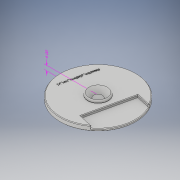
# Autodesk Inventor part: dissection_platform_v01
Saved by Autodesk Inventor 2019 (Build 230136000, 136)
## iProperties
Created: 2018-12-14
Part Number: dissection_platform_v01
Material: Generic
Document SubType Name: Modeling
Designer: Wilson Lab
Density: 1 g/cm^3
Appearance: Default
Author: Wilson Lab
Autodesk Inventor part; units mm, degrees
ref_plane "YZ Plane" through (0, 0, 0) normal (1, 0, 0) x (0, 1, 0)
ref_plane "XZ Plane" through (0, 0, 0) normal (0, 1, 0) x (-1, 0, 0)
ref_plane "XY Plane" through (0, 0, 0) normal (0, 0, 1) x (1, 0, 0)
sketch "Base Material Sketch" plane through (0, 0, 0) normal (0, 1, 0) x (-1, 0, 0)
  circle A0 centre (0, 0) radius 32.5
  dimension "d0" = 65
  constraints: 1 centre point, 1 coincident
  measures "d0" diameter of A0
extrude "Base Material Extrusion" add sketch "Base Material Sketch" along normal blind 4
sketch "Magnet Recess" plane through (0, 0, 0) normal (0, -1, 0) x (1, 0, 0)
  circle A0 centre (0, 0) radius 32.5 projected
  circle A1 centre (0, 27.5) radius 3.5
  line L0 (0, 0) -> (0, 32.5) construction
  circle A2 centre (0, 0) radius 32.5 construction
  circle A3 centre (-26.1541, 8.498) radius 3.5
  circle A4 centre (-16.1641, -22.248) radius 3.5
  circle A5 centre (16.1641, -22.248) radius 3.5
  circle A6 centre (26.1541, 8.498) radius 3.5
  dimension "d3" = 7
  dimension "d4" = 5
  dimension "d7" = 360
  constraints: 5 centre point, 2 end point, 1 point on line, 1 vertical, 1 vertical alignment, 12 other
  measures "d3" diameter of A1
  measures "d4" distance of A1.centre L0.end
extrude "Bottom Magnet Recess" cut sketch "Magnet Recess" against normal blind 1 contours A1 | A3 | A4 | A5 | A6
sketch "Central Well" plane through (0, 4, 0) normal (0, 1, 0) x (1, 0, 0)
  circle A0 centre (0, 0) radius 32.5 construction
  circle A1 centre (0, 0) radius 3.75
  dimension "d12" = 7.5
  constraints: 1 centre point, 1 coincident
  measures "d12" diameter of A1
extrude "Well Recess" cut sketch "Central Well" against normal blind 2
sketch "Sketch6" plane through (0, 4, 0) normal (0, 1, 0) x (1, 0, 0)
  circle A0 centre (0, 0) radius 7.75
  circle A1 centre (0, 0) radius 8.75
  dimension "d22" = 15.5
  dimension "d23" = 17.5
  constraints: 2 centre point, 2 coincident
  measures "d22" diameter of A0
  measures "d23" diameter of A1
extrude "Well Wall" add sketch "Sketch6" along normal blind 2
sketch "kimwipe recess sketch" plane through (0, 4, 0) normal (0, 1, 0) x (1, 0, 0)
  circle A0 centre (0, 0) radius 32.5 construction
  circle A1 centre (0, 0) radius 8.75 construction
  circle A2 centre (0, 0) radius 3.75 construction
  circle A3 centre (0, 0) radius 32.5 construction
  circle A4 centre (0, 0) radius 32.5 projected
  line L0 (16.9285, 17.1162) -> (55.4596, 8.4325)
  line L1 (55.4596, 8.4325) -> (46.4812, -31.4067)
  line L2 (46.4812, -31.4067) -> (7.95, -22.723)
  line L3 (7.95, -22.723) -> (16.9285, 17.1162)
  line L4 (16.9285, 17.1162) -> (46.4812, -31.4067) construction
  line L5 (55.4596, 8.4325) -> (7.95, -22.723) construction
  line L6 (0, 0) -> (12.4392, -2.8034) construction
  point P0 (31.7048, -7.1453)
  constraints: 14 end point, 3 midpoint, 2 parallel, 2 perpendicular, 1 coincident, 2 other
chamfer "Well Chamfer" distance 2 angle 45 2 edges at (-3.75, 4, 0) (-7.75, 4, 0)
fillet "Well Wall Fillet" radius 2 1 edges at (-8.75, 6, 0)
extrude "kimwipe recess" cut sketch "kimwipe recess sketch" against normal blind 2 contours A4 L2 L3 L0 | A4 L0 L1 L2 picked at (18.8525, -4.2886)
fillet "Aesthetic Filet" radius 0.5 14 edges at (12.6641, 0, -22.248) (-19.6641, 0, -22.248) (-29.6541, 0, 8.498) (-3.5, 0, 27.5) (22.6541, 0, 8.498) (32.5, 0, 0) (-7.3725, 4, -31.6527) (-14.1511, 4, 29.2574) (31.7048, 2, 7.1453) (12.4392, 4, 2.8034) (14.0633, 4, 24.1007) (20.1767, 3, 25.4785) (29.1551, 3, -14.3607) (23.0418, 4, -15.7384)
sketch "Sketch8" plane through (0, 4, 0) normal (0, 1, 0) x (-0.219854, 0, 0.9755328)
  line L0 (-23.8285, -62.331) -> (23.8285, -62.331) construction
  line L1 (23.8285, -62.331) -> (23.8285, 17.5) construction
  line L2 (23.8285, 17.5) -> (-23.8285, 17.5) construction
  line L3 (-23.8285, 17.5) -> (-23.8285, -62.331) construction
  circle A0 centre (0, 0) radius 17.5
  line L4 (-23.8285, 17.5) -> (23.8285, 17.5)
  line L5 (0, 0) -> (0, 17.5)
  line L6 (-14.128, -23.1128) -> (-14.3555, -23.1128)
  line L7 (-14.3555, -23.1128) -> (-14.3555, -22.9757)
  spline S0 degree 2 poles (-14.3555, -22.9757) (-14.408, -23.0194) (-14.4853, -23.0778) (-14.5378, -23.1026) knots 0 0 0 1 2 2 2
  spline S1 degree 2 poles (-14.5378, -23.1026) (-14.586, -23.1259) (-14.6895, -23.1507) (-14.7581, -23.1507) knots 0 0 0 1 2 2 2
  spline S2 degree 2 poles (-14.7581, -23.1507) (-14.869, -23.1507) (-15.0557, -23.0588) (-15.1213, -22.9698) knots 0 0 0 1 2 2 2
  spline S3 degree 2 poles (-15.1213, -22.9698) (-15.187, -22.8808) (-15.2599, -22.6183) (-15.2599, -22.4476) knots 0 0 0 1 2 2 2
  spline S4 degree 2 poles (-15.2599, -22.4476) (-15.2599, -22.2697) (-15.168, -22.01) (-15.0878, -21.9123) knots 0 0 0 1 2 2 2
  spline S5 degree 2 poles (-15.0878, -21.9123) (-15.0134, -21.8248) (-14.8048, -21.7241) (-14.6895, -21.7241) knots 0 0 0 1 2 2 2
  spline S6 degree 2 poles (-14.6895, -21.7241) (-14.5889, -21.7241) (-14.4387, -21.7693) (-14.3555, -21.816) knots 0 0 0 1 2 2 2
  line L8 (-14.3555, -21.816) -> (-14.3555, -21.2325)
  line L9 (-14.3555, -21.2325) -> (-14.128, -21.2325)
  line L10 (-14.128, -21.2325) -> (-14.128, -23.1128)
  line L11 (-14.3555, -22.7846) -> (-14.3555, -22.0042)
  spline S7 degree 2 poles (-14.3555, -22.0042) (-14.4401, -21.9633) (-14.5743, -21.9327) (-14.6516, -21.9327) knots 0 0 0 1 2 2 2
  spline S8 degree 2 poles (-14.6516, -21.9327) (-14.8267, -21.9327) (-15.025, -22.1953) (-15.025, -22.4432) knots 0 0 0 1 2 2 2
  spline S9 degree 2 poles (-15.025, -22.4432) (-15.025, -22.6825) (-14.8733, -22.9348) (-14.7056, -22.9348) knots 0 0 0 1 2 2 2
  spline S10 degree 2 poles (-14.7056, -22.9348) (-14.6166, -22.9348) (-14.4357, -22.8531) (-14.3555, -22.7846) knots 0 0 0 1 2 2 2
  line L12 (-13.5664, -23.1128) -> (-13.7939, -23.1128)
  line L13 (-13.7939, -23.1128) -> (-13.7939, -21.762)
  line L14 (-13.7939, -21.762) -> (-13.5664, -21.762)
  line L15 (-13.5664, -21.762) -> (-13.5664, -23.1128)
  line L16 (-13.5503, -21.5374) -> (-13.8085, -21.5374)
  line L17 (-13.8085, -21.5374) -> (-13.8085, -21.3011)
  line L18 (-13.8085, -21.3011) -> (-13.5503, -21.3011)
  line L19 (-13.5503, -21.3011) -> (-13.5503, -21.5374)
  spline S11 degree 2 poles (-12.8677, -23.1449) (-13.0033, -23.1449) (-13.2382, -23.0719) (-13.3155, -23.0311) knots 0 0 0 1 2 2 2
  line L20 (-13.3155, -23.0311) -> (-13.3155, -22.7758)
  line L21 (-13.3155, -22.7758) -> (-13.3038, -22.7758)
  spline S12 degree 2 poles (-13.3038, -22.7758) (-13.2746, -22.7992) (-13.1959, -22.8546) (-13.1302, -22.8852) knots 0 0 0 1 2 2 2
  spline S13 degree 2 poles (-13.1302, -22.8852) (-13.0733, -22.9129) (-12.9333, -22.9538) (-12.8589, -22.9538) knots 0 0 0 1 2 2 2
  spline S14 degree 2 poles (-12.8589, -22.9538) (-12.8049, -22.9538) (-12.681, -22.929) (-12.6518, -22.9086) knots 0 0 0 1 2 2 2
  spline S15 degree 2 poles (-12.6518, -22.9086) (-12.6095, -22.8808) (-12.5716, -22.8181) (-12.5716, -22.7539) knots 0 0 0 1 2 2 2
  spline S16 degree 2 poles (-12.5716, -22.7539) (-12.5716, -22.6737) (-12.6591, -22.5906) (-12.7714, -22.5628) knots 0 0 0 1 2 2 2
  spline S17 degree 2 poles (-12.7714, -22.5628) (-12.8152, -22.5526) (-12.9552, -22.5235) (-13.015, -22.5074) knots 0 0 0 1 2 2 2
  spline S18 degree 2 poles (-13.015, -22.5074) (-13.1696, -22.4622) (-13.3096, -22.2755) (-13.3096, -22.1427) knots 0 0 0 1 2 2 2
  spline S19 degree 2 poles (-13.3096, -22.1427) (-13.3096, -21.959) (-13.034, -21.7299) (-12.8064, -21.7299) knots 0 0 0 1 2 2 2
  spline S20 degree 2 poles (-12.8064, -21.7299) (-12.6941, -21.7299) (-12.4665, -21.7854) (-12.3892, -21.8277) knots 0 0 0 1 2 2 2
  line L22 (-12.3892, -21.8277) -> (-12.3892, -22.0713)
  line L23 (-12.3892, -22.0713) -> (-12.4009, -22.0713)
  spline S21 degree 2 poles (-12.4009, -22.0713) (-12.4884, -22.0013) (-12.7014, -21.921) (-12.8108, -21.921) knots 0 0 0 1 2 2 2
  spline S22 degree 2 poles (-12.8108, -21.921) (-12.9231, -21.921) (-13.0777, -22.0158) (-13.0777, -22.1107) knots 0 0 0 1 2 2 2
  spline S23 degree 2 poles (-13.0777, -22.1107) (-13.0777, -22.1967) (-12.9858, -22.2799) (-12.8837, -22.3061) knots 0 0 0 1 2 2 2
  spline S24 degree 2 poles (-12.8837, -22.3061) (-12.8341, -22.3192) (-12.7087, -22.3455) (-12.6401, -22.3616) knots 0 0 0 1 2 2 2
  spline S25 degree 2 poles (-12.6401, -22.3616) (-12.4913, -22.3995) (-12.3396, -22.5731) (-12.3396, -22.7233) knots 0 0 0 1 2 2 2
  spline S26 degree 2 poles (-12.3396, -22.7233) (-12.3396, -22.8108) (-12.4082, -22.9654) (-12.4753, -23.0223) knots 0 0 0 1 2 2 2
  spline S27 degree 2 poles (-12.4753, -23.0223) (-12.5468, -23.0821) (-12.7291, -23.1449) (-12.8677, -23.1449) knots 0 0 0 1 2 2 2
  spline S28 degree 2 poles (-11.7635, -23.1449) (-11.8991, -23.1449) (-12.134, -23.0719) (-12.2113, -23.0311) knots 0 0 0 1 2 2 2
  line L24 (-12.2113, -23.0311) -> (-12.2113, -22.7758)
  line L25 (-12.2113, -22.7758) -> (-12.1996, -22.7758)
  spline S29 degree 2 poles (-12.1996, -22.7758) (-12.1704, -22.7992) (-12.0917, -22.8546) (-12.026, -22.8852) knots 0 0 0 1 2 2 2
  spline S30 degree 2 poles (-12.026, -22.8852) (-11.9691, -22.9129) (-11.8291, -22.9538) (-11.7547, -22.9538) knots 0 0 0 1 2 2 2
  spline S31 degree 2 poles (-11.7547, -22.9538) (-11.7007, -22.9538) (-11.5767, -22.929) (-11.5476, -22.9086) knots 0 0 0 1 2 2 2
  spline S32 degree 2 poles (-11.5476, -22.9086) (-11.5053, -22.8808) (-11.4673, -22.8181) (-11.4673, -22.7539) knots 0 0 0 1 2 2 2
  spline S33 degree 2 poles (-11.4673, -22.7539) (-11.4673, -22.6737) (-11.5549, -22.5906) (-11.6672, -22.5628) knots 0 0 0 1 2 2 2
  spline S34 degree 2 poles (-11.6672, -22.5628) (-11.7109, -22.5526) (-11.851, -22.5235) (-11.9108, -22.5074) knots 0 0 0 1 2 2 2
  spline S35 degree 2 poles (-11.9108, -22.5074) (-12.0654, -22.4622) (-12.2054, -22.2755) (-12.2054, -22.1427) knots 0 0 0 1 2 2 2
  spline S36 degree 2 poles (-12.2054, -22.1427) (-12.2054, -21.959) (-11.9297, -21.7299) (-11.7022, -21.7299) knots 0 0 0 1 2 2 2
  spline S37 degree 2 poles (-11.7022, -21.7299) (-11.5899, -21.7299) (-11.3623, -21.7854) (-11.285, -21.8277) knots 0 0 0 1 2 2 2
  line L26 (-11.285, -21.8277) -> (-11.285, -22.0713)
  line L27 (-11.285, -22.0713) -> (-11.2967, -22.0713)
  spline S38 degree 2 poles (-11.2967, -22.0713) (-11.3842, -22.0013) (-11.5972, -21.921) (-11.7066, -21.921) knots 0 0 0 1 2 2 2
  spline S39 degree 2 poles (-11.7066, -21.921) (-11.8189, -21.921) (-11.9735, -22.0158) (-11.9735, -22.1107) knots 0 0 0 1 2 2 2
  spline S40 degree 2 poles (-11.9735, -22.1107) (-11.9735, -22.1967) (-11.8816, -22.2799) (-11.7795, -22.3061) knots 0 0 0 1 2 2 2
  spline S41 degree 2 poles (-11.7795, -22.3061) (-11.7299, -22.3192) (-11.6045, -22.3455) (-11.5359, -22.3616) knots 0 0 0 1 2 2 2
  spline S42 degree 2 poles (-11.5359, -22.3616) (-11.3871, -22.3995) (-11.2354, -22.5731) (-11.2354, -22.7233) knots 0 0 0 1 2 2 2
  spline S43 degree 2 poles (-11.2354, -22.7233) (-11.2354, -22.8108) (-11.304, -22.9654) (-11.3711, -23.0223) knots 0 0 0 1 2 2 2
  spline S44 degree 2 poles (-11.3711, -23.0223) (-11.4425, -23.0821) (-11.6249, -23.1449) (-11.7635, -23.1449) knots 0 0 0 1 2 2 2
  spline S45 degree 2 poles (-10.4375, -23.1434) (-10.7613, -23.1434) (-11.1173, -22.7802) (-11.1173, -22.4447) knots 0 0 0 1 2 2 2
  spline S46 degree 2 poles (-11.1173, -22.4447) (-11.1173, -22.115) (-10.7716, -21.7241) (-10.4929, -21.7241) knots 0 0 0 1 2 2 2
  spline S47 degree 2 poles (-10.4929, -21.7241) (-10.3675, -21.7241) (-10.1735, -21.797) (-10.102, -21.8744) knots 0 0 0 1 2 2 2
  spline S48 degree 2 poles (-10.102, -21.8744) (-10.0291, -21.9517) (-9.9518, -22.1748) (-9.9518, -22.3368) knots 0 0 0 1 2 2 2
  line L28 (-9.9518, -22.3368) -> (-9.9518, -22.4607)
  line L29 (-9.9518, -22.4607) -> (-10.8868, -22.4607)
  spline S49 degree 2 poles (-10.8868, -22.4607) (-10.8868, -22.6956) (-10.6505, -22.945) (-10.4404, -22.945) knots 0 0 0 1 2 2 2
  spline S50 degree 2 poles (-10.4404, -22.945) (-10.366, -22.945) (-10.2216, -22.9115) (-10.1633, -22.8852) knots 0 0 0 1 2 2 2
  spline S51 degree 2 poles (-10.1633, -22.8852) (-10.102, -22.856) (-10.0174, -22.805) (-9.9897, -22.7816) knots 0 0 0 1 2 2 2
  line L30 (-9.9897, -22.7816) -> (-9.9766, -22.7816)
  line L31 (-9.9766, -22.7816) -> (-9.9766, -23.0296)
  spline S52 degree 2 poles (-9.9766, -23.0296) (-10.016, -23.0457) (-10.1356, -23.0923) (-10.1823, -23.1055) knots 0 0 0 1 2 2 2
  spline S53 degree 2 poles (-10.1823, -23.1055) (-10.2479, -23.1244) (-10.3558, -23.1434) (-10.4375, -23.1434) knots 0 0 0 1 2 2 2
  spline S54 degree 2 poles (-10.1735, -22.2872) (-10.1764, -22.1953) (-10.2143, -22.0611) (-10.2508, -22.0158) knots 0 0 0 1 2 2 2
  spline S55 degree 2 poles (-10.2508, -22.0158) (-10.2902, -21.9648) (-10.4142, -21.9108) (-10.5061, -21.9108) knots 0 0 0 1 2 2 2
  spline S56 degree 2 poles (-10.5061, -21.9108) (-10.5965, -21.9108) (-10.7234, -21.9648) (-10.7759, -22.0173) knots 0 0 0 1 2 2 2
  spline S57 degree 2 poles (-10.7759, -22.0173) (-10.827, -22.0713) (-10.8795, -22.2011) (-10.8868, -22.2872) knots 0 0 0 1 2 2 2
  line L32 (-10.8868, -22.2872) -> (-10.1735, -22.2872)
  spline S58 degree 2 poles (-9.1845, -23.1434) (-9.3246, -23.1434) (-9.5565, -23.0573) (-9.6396, -22.9698) knots 0 0 0 1 2 2 2
  spline S59 degree 2 poles (-9.6396, -22.9698) (-9.7228, -22.8838) (-9.8147, -22.6183) (-9.8147, -22.4403) knots 0 0 0 1 2 2 2
  spline S60 degree 2 poles (-9.8147, -22.4403) (-9.8147, -22.2624) (-9.7199, -22.0027) (-9.6396, -21.9152) knots 0 0 0 1 2 2 2
  spline S61 degree 2 poles (-9.6396, -21.9152) (-9.5594, -21.8262) (-9.3216, -21.7314) (-9.1845, -21.7314) knots 0 0 0 1 2 2 2
  spline S62 degree 2 poles (-9.1845, -21.7314) (-9.0737, -21.7314) (-8.8665, -21.7941) (-8.7863, -21.835) knots 0 0 0 1 2 2 2
  line L33 (-8.7863, -21.835) -> (-8.7863, -22.0902)
  line L34 (-8.7863, -22.0902) -> (-8.7994, -22.0902)
  spline S63 degree 2 poles (-8.7994, -22.0902) (-8.8242, -22.0698) (-8.9001, -22.0173) (-8.9541, -21.9896) knots 0 0 0 1 2 2 2
  spline S64 degree 2 poles (-8.9541, -21.9896) (-9.0022, -21.9663) (-9.1306, -21.9298) (-9.1889, -21.9298) knots 0 0 0 1 2 2 2
  spline S65 degree 2 poles (-9.1889, -21.9298) (-9.3654, -21.9298) (-9.5798, -22.1967) (-9.5798, -22.4403) knots 0 0 0 1 2 2 2
  spline S66 degree 2 poles (-9.5798, -22.4403) (-9.5798, -22.6781) (-9.3727, -22.945) (-9.1889, -22.945) knots 0 0 0 1 2 2 2
  spline S67 degree 2 poles (-9.1889, -22.945) (-9.078, -22.945) (-8.8767, -22.8531) (-8.7994, -22.7816) knots 0 0 0 1 2 2 2
  line L35 (-8.7994, -22.7816) -> (-8.7863, -22.7816)
  line L36 (-8.7863, -22.7816) -> (-8.7863, -23.0369)
  spline S68 degree 2 poles (-8.7863, -23.0369) (-8.8199, -23.053) (-8.922, -23.0982) (-8.9628, -23.1084) knots 0 0 0 1 2 2 2
  spline S69 degree 2 poles (-8.9628, -23.1084) (-9.0212, -23.1259) (-9.113, -23.1434) (-9.1845, -23.1434) knots 0 0 0 1 2 2 2
  spline S70 degree 2 poles (-8.1707, -23.139) (-8.356, -23.139) (-8.5646, -22.9275) (-8.5646, -22.6985) knots 0 0 0 1 2 2 2
  line L37 (-8.5646, -22.6985) -> (-8.5646, -21.9502)
  line L38 (-8.5646, -21.9502) -> (-8.7177, -21.9502)
  line L39 (-8.7177, -21.9502) -> (-8.7177, -21.762)
  line L40 (-8.7177, -21.762) -> (-8.5646, -21.762)
  line L41 (-8.5646, -21.762) -> (-8.5646, -21.374)
  line L42 (-8.5646, -21.374) -> (-8.337, -21.374)
  line L43 (-8.337, -21.374) -> (-8.337, -21.762)
  line L44 (-8.337, -21.762) -> (-7.9184, -21.762)
  line L45 (-7.9184, -21.762) -> (-7.9184, -21.9502)
  line L46 (-7.9184, -21.9502) -> (-8.337, -21.9502)
  line L47 (-8.337, -21.9502) -> (-8.337, -22.5935)
  spline S71 degree 2 poles (-8.337, -22.5935) (-8.337, -22.6956) (-8.3297, -22.8079) (-8.3049, -22.856) knots 0 0 0 1 2 2 2
  spline S72 degree 2 poles (-8.3049, -22.856) (-8.2845, -22.8983) (-8.1926, -22.9406) (-8.1139, -22.9406) knots 0 0 0 1 2 2 2
  spline S73 degree 2 poles (-8.1139, -22.9406) (-8.0584, -22.9406) (-7.9549, -22.9071) (-7.9315, -22.8969) knots 0 0 0 1 2 2 2
  line L48 (-7.9315, -22.8969) -> (-7.9184, -22.8969)
  line L49 (-7.9184, -22.8969) -> (-7.9184, -23.1011)
  spline S74 degree 2 poles (-7.9184, -23.1011) (-7.9826, -23.1186) (-8.1139, -23.139) (-8.1707, -23.139) knots 0 0 0 1 2 2 2
  line L50 (-7.5187, -23.1128) -> (-7.7463, -23.1128)
  line L51 (-7.7463, -23.1128) -> (-7.7463, -21.762)
  line L52 (-7.7463, -21.762) -> (-7.5187, -21.762)
  line L53 (-7.5187, -21.762) -> (-7.5187, -23.1128)
  line L54 (-7.5027, -21.5374) -> (-7.7609, -21.5374)
  line L55 (-7.7609, -21.5374) -> (-7.7609, -21.3011)
  line L56 (-7.7609, -21.3011) -> (-7.5027, -21.3011)
  line L57 (-7.5027, -21.3011) -> (-7.5027, -21.5374)
  spline S75 degree 2 poles (-6.0746, -22.4374) (-6.0746, -22.7787) (-6.4028, -23.1507) (-6.6771, -23.1507) knots 0 0 0 1 2 2 2
  spline S76 degree 2 poles (-6.6771, -23.1507) (-6.9586, -23.1507) (-7.281, -22.7671) (-7.281, -22.4374) knots 0 0 0 1 2 2 2
  spline S77 degree 2 poles (-7.281, -22.4374) (-7.281, -22.099) (-6.9484, -21.7241) (-6.6771, -21.7241) knots 0 0 0 1 2 2 2
  spline S78 degree 2 poles (-6.6771, -21.7241) (-6.4028, -21.7241) (-6.0746, -22.0975) (-6.0746, -22.4374) knots 0 0 0 1 2 2 2
  spline S79 degree 2 poles (-6.3095, -22.4374) (-6.3095, -22.1748) (-6.5006, -21.9196) (-6.6771, -21.9196) knots 0 0 0 1 2 2 2
  spline S80 degree 2 poles (-6.6771, -21.9196) (-6.8536, -21.9196) (-7.0461, -22.1748) (-7.0461, -22.4374) knots 0 0 0 1 2 2 2
  spline S81 degree 2 poles (-7.0461, -22.4374) (-7.0461, -22.6927) (-6.8536, -22.9552) (-6.6771, -22.9552) knots 0 0 0 1 2 2 2
  spline S82 degree 2 poles (-6.6771, -22.9552) (-6.502, -22.9552) (-6.3095, -22.697) (-6.3095, -22.4374) knots 0 0 0 1 2 2 2
  line L58 (-4.7808, -23.1128) -> (-5.0083, -23.1128)
  line L59 (-5.0083, -23.1128) -> (-5.0083, -22.3426)
  spline S83 degree 2 poles (-5.0083, -22.3426) (-5.0083, -22.2492) (-5.0259, -22.0888) (-5.0521, -22.0406) knots 0 0 0 1 2 2 2
  spline S84 degree 2 poles (-5.0521, -22.0406) (-5.0798, -21.9896) (-5.179, -21.94) (-5.2636, -21.94) knots 0 0 0 1 2 2 2
  spline S85 degree 2 poles (-5.2636, -21.94) (-5.3482, -21.94) (-5.5276, -22.0304) (-5.6137, -22.1034) knots 0 0 0 1 2 2 2
  line L60 (-5.6137, -22.1034) -> (-5.6137, -23.1128)
  line L61 (-5.6137, -23.1128) -> (-5.8412, -23.1128)
  line L62 (-5.8412, -23.1128) -> (-5.8412, -21.762)
  line L63 (-5.8412, -21.762) -> (-5.6137, -21.762)
  line L64 (-5.6137, -21.762) -> (-5.6137, -21.9123)
  spline S86 degree 2 poles (-5.6137, -21.9123) (-5.5116, -21.8204) (-5.3147, -21.7241) (-5.2038, -21.7241) knots 0 0 0 1 2 2 2
  spline S87 degree 2 poles (-5.2038, -21.7241) (-5.0054, -21.7241) (-4.7808, -21.9867) (-4.7808, -22.2361) knots 0 0 0 1 2 2 2
  line L65 (-4.7808, -22.2361) -> (-4.7808, -23.1128)
  line L66 (-3.2565, -23.4745) -> (-4.6451, -23.4745)
  line L67 (-4.6451, -23.4745) -> (-4.6451, -23.3184)
  line L68 (-4.6451, -23.3184) -> (-3.2565, -23.3184)
  line L69 (-3.2565, -23.3184) -> (-3.2565, -23.4745)
  spline S88 degree 2 poles (-1.9787, -22.4009) (-1.9787, -22.7393) (-2.3011, -23.139) (-2.5476, -23.139) knots 0 0 0 1 2 2 2
  spline S89 degree 2 poles (-2.5476, -23.139) (-2.6482, -23.139) (-2.8028, -23.0923) (-2.8831, -23.0442) knots 0 0 0 1 2 2 2
  line L70 (-2.8831, -23.0442) -> (-2.8831, -23.6102)
  line L71 (-2.8831, -23.6102) -> (-3.1106, -23.6102)
  line L72 (-3.1106, -23.6102) -> (-3.1106, -21.762)
  line L73 (-3.1106, -21.762) -> (-2.8831, -21.762)
  line L74 (-2.8831, -21.762) -> (-2.8831, -21.9035)
  spline S90 degree 2 poles (-2.8831, -21.9035) (-2.7985, -21.8262) (-2.5913, -21.7241) (-2.4703, -21.7241) knots 0 0 0 1 2 2 2
  spline S91 degree 2 poles (-2.4703, -21.7241) (-2.2383, -21.7241) (-1.9787, -22.0917) (-1.9787, -22.4009) knots 0 0 0 1 2 2 2
  spline S92 degree 2 poles (-2.2135, -22.4272) (-2.2135, -22.1953) (-2.3609, -21.94) (-2.5257, -21.94) knots 0 0 0 1 2 2 2
  spline S93 degree 2 poles (-2.5257, -21.94) (-2.622, -21.94) (-2.8028, -22.0261) (-2.8831, -22.0932) knots 0 0 0 1 2 2 2
  line L75 (-2.8831, -22.0932) -> (-2.8831, -22.8604)
  spline S94 degree 2 poles (-2.8831, -22.8604) (-2.7941, -22.9027) (-2.6672, -22.9348) (-2.5855, -22.9348) knots 0 0 0 1 2 2 2
  spline S95 degree 2 poles (-2.5855, -22.9348) (-2.409, -22.9348) (-2.2135, -22.6752) (-2.2135, -22.4272) knots 0 0 0 1 2 2 2
  line L76 (-1.5105, -23.1128) -> (-1.738, -23.1128)
  line L77 (-1.738, -23.1128) -> (-1.738, -21.2325)
  line L78 (-1.738, -21.2325) -> (-1.5105, -21.2325)
  line L79 (-1.5105, -21.2325) -> (-1.5105, -23.1128)
  spline S96 degree 2 poles (-0.4237, -22.9698) (-0.4515, -22.9902) (-0.5448, -23.0632) (-0.5886, -23.0851) knots 0 0 0 1 2 2 2
  spline S97 degree 2 poles (-0.5886, -23.0851) (-0.6484, -23.1171) (-0.7607, -23.1507) (-0.8628, -23.1507) knots 0 0 0 1 2 2 2
  spline S98 degree 2 poles (-0.8628, -23.1507) (-0.9459, -23.1507) (-1.0962, -23.088) (-1.1531, -23.0311) knots 0 0 0 1 2 2 2
  spline S99 degree 2 poles (-1.1531, -23.0311) (-1.207, -22.9757) (-1.2727, -22.8123) (-1.2727, -22.7218) knots 0 0 0 1 2 2 2
  spline S100 degree 2 poles (-1.2727, -22.7218) (-1.2727, -22.5818) (-1.1545, -22.3834) (-1.0262, -22.3265) knots 0 0 0 1 2 2 2
  spline S101 degree 2 poles (-1.0262, -22.3265) (-0.9124, -22.274) (-0.6032, -22.2346) (-0.4237, -22.2244) knots 0 0 0 1 2 2 2
  line L80 (-0.4237, -22.2244) -> (-0.4237, -22.1807)
  spline S102 degree 2 poles (-0.4237, -22.1807) (-0.4237, -22.1019) (-0.4719, -22.0042) (-0.5156, -21.9765) knots 0 0 0 1 2 2 2
  spline S103 degree 2 poles (-0.5156, -21.9765) (-0.5594, -21.9487) (-0.6848, -21.9312) (-0.7519, -21.9312) knots 0 0 0 1 2 2 2
  spline S104 degree 2 poles (-0.7519, -21.9312) (-0.8307, -21.9312) (-1.0437, -21.9779) (-1.1502, -22.0231) knots 0 0 0 1 2 2 2
  line L81 (-1.1502, -22.0231) -> (-1.1633, -22.0231)
  line L82 (-1.1633, -22.0231) -> (-1.1633, -21.7912)
  spline S105 degree 2 poles (-1.1633, -21.7912) (-1.1006, -21.7737) (-0.8657, -21.7299) (-0.7505, -21.7299) knots 0 0 0 1 2 2 2
  spline S106 degree 2 poles (-0.7505, -21.7299) (-0.6105, -21.7299) (-0.4194, -21.7737) (-0.3435, -21.8306) knots 0 0 0 1 2 2 2
  spline S107 degree 2 poles (-0.3435, -21.8306) (-0.2691, -21.886) (-0.1962, -22.0625) (-0.1962, -22.1894) knots 0 0 0 1 2 2 2
  line L83 (-0.1962, -22.1894) -> (-0.1962, -23.1128)
  line L84 (-0.1962, -23.1128) -> (-0.4237, -23.1128)
  line L85 (-0.4237, -23.1128) -> (-0.4237, -22.9698)
  line L86 (-0.4237, -22.7802) -> (-0.4237, -22.4053)
  spline S108 degree 2 poles (-0.4237, -22.4053) (-0.5054, -22.4126) (-0.7519, -22.4374) (-0.8293, -22.4607) knots 0 0 0 1 2 2 2
  spline S109 degree 2 poles (-0.8293, -22.4607) (-0.9197, -22.4885) (-1.0378, -22.6037) (-1.0378, -22.7058) knots 0 0 0 1 2 2 2
  spline S110 degree 2 poles (-1.0378, -22.7058) (-1.0378, -22.8225) (-0.9066, -22.9406) (-0.7811, -22.9406) knots 0 0 0 1 2 2 2
  spline S111 degree 2 poles (-0.7811, -22.9406) (-0.6746, -22.9406) (-0.4996, -22.8487) (-0.4237, -22.7802) knots 0 0 0 1 2 2 2
  spline S112 degree 2 poles (0.5317, -23.139) (0.3464, -23.139) (0.1378, -22.9275) (0.1378, -22.6985) knots 0 0 0 1 2 2 2
  line L87 (0.1378, -22.6985) -> (0.1378, -21.9502)
  line L88 (0.1378, -21.9502) -> (-0.0153, -21.9502)
  line L89 (-0.0153, -21.9502) -> (-0.0153, -21.762)
  line L90 (-0.0153, -21.762) -> (0.1378, -21.762)
  line L91 (0.1378, -21.762) -> (0.1378, -21.374)
  line L92 (0.1378, -21.374) -> (0.3654, -21.374)
  line L93 (0.3654, -21.374) -> (0.3654, -21.762)
  line L94 (0.3654, -21.762) -> (0.784, -21.762)
  line L95 (0.784, -21.762) -> (0.784, -21.9502)
  line L96 (0.784, -21.9502) -> (0.3654, -21.9502)
  line L97 (0.3654, -21.9502) -> (0.3654, -22.5935)
  spline S113 degree 2 poles (0.3654, -22.5935) (0.3654, -22.6956) (0.3727, -22.8079) (0.3975, -22.856) knots 0 0 0 1 2 2 2
  spline S114 degree 2 poles (0.3975, -22.856) (0.4179, -22.8983) (0.5098, -22.9406) (0.5886, -22.9406) knots 0 0 0 1 2 2 2
  spline S115 degree 2 poles (0.5886, -22.9406) (0.644, -22.9406) (0.7476, -22.9071) (0.7709, -22.8969) knots 0 0 0 1 2 2 2
  line L98 (0.7709, -22.8969) -> (0.784, -22.8969)
  line L99 (0.784, -22.8969) -> (0.784, -23.1011)
  spline S116 degree 2 poles (0.784, -23.1011) (0.7199, -23.1186) (0.5886, -23.139) (0.5317, -23.139) knots 0 0 0 1 2 2 2
  line L100 (1.6622, -21.4513) -> (1.6505, -21.4513)
  spline S117 degree 2 poles (1.6505, -21.4513) (1.6199, -21.4397) (1.5061, -21.4192) (1.4609, -21.4192) knots 0 0 0 1 2 2 2
  spline S118 degree 2 poles (1.4609, -21.4192) (1.3179, -21.4192) (1.1954, -21.5476) (1.1954, -21.7168) knots 0 0 0 1 2 2 2
  line L101 (1.1954, -21.7168) -> (1.1954, -21.762)
  line L102 (1.1954, -21.762) -> (1.5717, -21.762)
  line L103 (1.5717, -21.762) -> (1.5717, -21.9502)
  line L104 (1.5717, -21.9502) -> (1.2027, -21.9502)
  line L105 (1.2027, -21.9502) -> (1.2027, -23.1128)
  line L106 (1.2027, -23.1128) -> (0.9751, -23.1128)
  line L107 (0.9751, -23.1128) -> (0.9751, -21.9502)
  line L108 (0.9751, -21.9502) -> (0.822, -21.9502)
  line L109 (0.822, -21.9502) -> (0.822, -21.762)
  line L110 (0.822, -21.762) -> (0.9751, -21.762)
  line L111 (0.9751, -21.762) -> (0.9751, -21.7168)
  spline S119 degree 2 poles (0.9751, -21.7168) (0.9751, -21.4747) (1.21, -21.2209) (1.4288, -21.2209) knots 0 0 0 1 2 2 2
  spline S120 degree 2 poles (1.4288, -21.2209) (1.4915, -21.2209) (1.6126, -21.234) (1.6622, -21.2427) knots 0 0 0 1 2 2 2
  line L112 (1.6622, -21.2427) -> (1.6622, -21.4513)
  spline S121 degree 2 poles (2.8495, -22.4374) (2.8495, -22.7787) (2.5213, -23.1507) (2.2471, -23.1507) knots 0 0 0 1 2 2 2
  spline S122 degree 2 poles (2.2471, -23.1507) (1.9656, -23.1507) (1.6432, -22.7671) (1.6432, -22.4374) knots 0 0 0 1 2 2 2
  spline S123 degree 2 poles (1.6432, -22.4374) (1.6432, -22.099) (1.9758, -21.7241) (2.2471, -21.7241) knots 0 0 0 1 2 2 2
  spline S124 degree 2 poles (2.2471, -21.7241) (2.5213, -21.7241) (2.8495, -22.0975) (2.8495, -22.4374) knots 0 0 0 1 2 2 2
  spline S125 degree 2 poles (2.6147, -22.4374) (2.6147, -22.1748) (2.4236, -21.9196) (2.2471, -21.9196) knots 0 0 0 1 2 2 2
  spline S126 degree 2 poles (2.2471, -21.9196) (2.0706, -21.9196) (1.878, -22.1748) (1.878, -22.4374) knots 0 0 0 1 2 2 2
  spline S127 degree 2 poles (1.878, -22.4374) (1.878, -22.6927) (2.0706, -22.9552) (2.2471, -22.9552) knots 0 0 0 1 2 2 2
  spline S128 degree 2 poles (2.2471, -22.9552) (2.4221, -22.9552) (2.6147, -22.697) (2.6147, -22.4374) knots 0 0 0 1 2 2 2
  line L113 (3.7991, -22.0056) -> (3.7874, -22.0056)
  spline S129 degree 2 poles (3.7874, -22.0056) (3.7612, -21.9983) (3.7043, -21.9954) (3.6649, -21.9954) knots 0 0 0 1 2 2 2
  spline S130 degree 2 poles (3.6649, -21.9954) (3.573, -21.9954) (3.3921, -22.0757) (3.3105, -22.1544) knots 0 0 0 1 2 2 2
  line L114 (3.3105, -22.1544) -> (3.3105, -23.1128)
  line L115 (3.3105, -23.1128) -> (3.0829, -23.1128)
  line L116 (3.0829, -23.1128) -> (3.0829, -21.762)
  line L117 (3.0829, -21.762) -> (3.3105, -21.762)
  line L118 (3.3105, -21.762) -> (3.3105, -21.9633)
  spline S131 degree 2 poles (3.3105, -21.9633) (3.4344, -21.8525) (3.6197, -21.762) (3.7072, -21.762) knots 0 0 0 1 2 2 2
  spline S132 degree 2 poles (3.7072, -21.762) (3.7422, -21.762) (3.7772, -21.765) (3.7991, -21.7693) knots 0 0 0 1 2 2 2
  line L119 (3.7991, -21.7693) -> (3.7991, -22.0056)
  line L120 (5.5072, -23.1128) -> (5.5072, -22.3309)
  spline S133 degree 2 poles (5.5072, -22.3309) (5.5072, -22.2376) (5.4926, -22.0786) (5.4693, -22.0348) knots 0 0 0 1 2 2 2
  spline S134 degree 2 poles (5.4693, -22.0348) (5.4459, -21.9867) (5.357, -21.94) (5.2797, -21.94) knots 0 0 0 1 2 2 2
  spline S135 degree 2 poles (5.2797, -21.94) (5.2096, -21.94) (5.0492, -22.0261) (4.9646, -22.1077) knots 0 0 0 1 2 2 2
  spline S136 degree 2 poles (4.9646, -22.1077) (4.966, -22.1282) (4.969, -22.1851) (4.969, -22.223) knots 0 0 0 1 2 2 2
  line L121 (4.969, -22.223) -> (4.969, -23.1128)
  line L122 (4.969, -23.1128) -> (4.7414, -23.1128)
  line L123 (4.7414, -23.1128) -> (4.7414, -22.3309)
  spline S137 degree 2 poles (4.7414, -22.3309) (4.7414, -22.2376) (4.7268, -22.0786) (4.7035, -22.0348) knots 0 0 0 1 2 2 2
  spline S138 degree 2 poles (4.7035, -22.0348) (4.6801, -21.9867) (4.5912, -21.94) (4.5139, -21.94) knots 0 0 0 1 2 2 2
  spline S139 degree 2 poles (4.5139, -21.94) (4.4409, -21.94) (4.279, -22.0319) (4.2032, -22.1034) knots 0 0 0 1 2 2 2
  line L124 (4.2032, -22.1034) -> (4.2032, -23.1128)
  line L125 (4.2032, -23.1128) -> (3.9756, -23.1128)
  line L126 (3.9756, -23.1128) -> (3.9756, -21.762)
  line L127 (3.9756, -21.762) -> (4.2032, -21.762)
  line L128 (4.2032, -21.762) -> (4.2032, -21.9108)
  spline S140 degree 2 poles (4.2032, -21.9108) (4.2921, -21.8218) (4.4672, -21.7241) (4.5722, -21.7241) knots 0 0 0 1 2 2 2
  spline S141 degree 2 poles (4.5722, -21.7241) (4.6918, -21.7241) (4.8771, -21.8335) (4.9252, -21.9575) knots 0 0 0 1 2 2 2
  spline S142 degree 2 poles (4.9252, -21.9575) (5.0288, -21.8423) (5.2242, -21.7241) (5.338, -21.7241) knots 0 0 0 1 2 2 2
  spline S143 degree 2 poles (5.338, -21.7241) (5.4255, -21.7241) (5.5685, -21.7781) (5.621, -21.8393) knots 0 0 0 1 2 2 2
  spline S144 degree 2 poles (5.621, -21.8393) (5.675, -21.9006) (5.7348, -22.0844) (5.7348, -22.223) knots 0 0 0 1 2 2 2
  line L129 (5.7348, -22.223) -> (5.7348, -23.1128)
  line L130 (5.7348, -23.1128) -> (5.5072, -23.1128)
  line L131 (7.2591, -23.4745) -> (5.8704, -23.4745)
  line L132 (5.8704, -23.4745) -> (5.8704, -23.3184)
  line L133 (5.8704, -23.3184) -> (7.2591, -23.3184)
  line L134 (7.2591, -23.3184) -> (7.2591, -23.4745)
  line L135 (8.9365, -23.1128) -> (8.9365, -22.3309)
  spline S145 degree 2 poles (8.9365, -22.3309) (8.9365, -22.2376) (8.922, -22.0786) (8.8986, -22.0348) knots 0 0 0 1 2 2 2
  spline S146 degree 2 poles (8.8986, -22.0348) (8.8753, -21.9867) (8.7863, -21.94) (8.709, -21.94) knots 0 0 0 1 2 2 2
  spline S147 degree 2 poles (8.709, -21.94) (8.639, -21.94) (8.4785, -22.0261) (8.3939, -22.1077) knots 0 0 0 1 2 2 2
  spline S148 degree 2 poles (8.3939, -22.1077) (8.3954, -22.1282) (8.3983, -22.1851) (8.3983, -22.223) knots 0 0 0 1 2 2 2
  line L136 (8.3983, -22.223) -> (8.3983, -23.1128)
  line L137 (8.3983, -23.1128) -> (8.1707, -23.1128)
  line L138 (8.1707, -23.1128) -> (8.1707, -22.3309)
  spline S149 degree 2 poles (8.1707, -22.3309) (8.1707, -22.2376) (8.1562, -22.0786) (8.1328, -22.0348) knots 0 0 0 1 2 2 2
  spline S150 degree 2 poles (8.1328, -22.0348) (8.1095, -21.9867) (8.0205, -21.94) (7.9432, -21.94) knots 0 0 0 1 2 2 2
  spline S151 degree 2 poles (7.9432, -21.94) (7.8703, -21.94) (7.7083, -22.0319) (7.6325, -22.1034) knots 0 0 0 1 2 2 2
  line L139 (7.6325, -22.1034) -> (7.6325, -23.1128)
  line L140 (7.6325, -23.1128) -> (7.4049, -23.1128)
  line L141 (7.4049, -23.1128) -> (7.4049, -21.762)
  line L142 (7.4049, -21.762) -> (7.6325, -21.762)
  line L143 (7.6325, -21.762) -> (7.6325, -21.9108)
  spline S152 degree 2 poles (7.6325, -21.9108) (7.7215, -21.8218) (7.8965, -21.7241) (8.0015, -21.7241) knots 0 0 0 1 2 2 2
  spline S153 degree 2 poles (8.0015, -21.7241) (8.1212, -21.7241) (8.3064, -21.8335) (8.3545, -21.9575) knots 0 0 0 1 2 2 2
  spline S154 degree 2 poles (8.3545, -21.9575) (8.4581, -21.8423) (8.6536, -21.7241) (8.7673, -21.7241) knots 0 0 0 1 2 2 2
  spline S155 degree 2 poles (8.7673, -21.7241) (8.8549, -21.7241) (8.9978, -21.7781) (9.0503, -21.8393) knots 0 0 0 1 2 2 2
  spline S156 degree 2 poles (9.0503, -21.8393) (9.1043, -21.9006) (9.1641, -22.0844) (9.1641, -22.223) knots 0 0 0 1 2 2 2
  line L144 (9.1641, -22.223) -> (9.1641, -23.1128)
  line L145 (9.1641, -23.1128) -> (8.9365, -23.1128)
  line L146 (11.0152, -23.1128) -> (11.0152, -22.3309)
  spline S157 degree 2 poles (11.0152, -22.3309) (11.0152, -22.2376) (11.0006, -22.0786) (10.9772, -22.0348) knots 0 0 0 1 2 2 2
  spline S158 degree 2 poles (10.9772, -22.0348) (10.9539, -21.9867) (10.8649, -21.94) (10.7876, -21.94) knots 0 0 0 1 2 2 2
  spline S159 degree 2 poles (10.7876, -21.94) (10.7176, -21.94) (10.5571, -22.0261) (10.4725, -22.1077) knots 0 0 0 1 2 2 2
  spline S160 degree 2 poles (10.4725, -22.1077) (10.474, -22.1282) (10.4769, -22.1851) (10.4769, -22.223) knots 0 0 0 1 2 2 2
  line L147 (10.4769, -22.223) -> (10.4769, -23.1128)
  line L148 (10.4769, -23.1128) -> (10.2494, -23.1128)
  line L149 (10.2494, -23.1128) -> (10.2494, -22.3309)
  spline S161 degree 2 poles (10.2494, -22.3309) (10.2494, -22.2376) (10.2348, -22.0786) (10.2114, -22.0348) knots 0 0 0 1 2 2 2
  spline S162 degree 2 poles (10.2114, -22.0348) (10.1881, -21.9867) (10.0991, -21.94) (10.0218, -21.94) knots 0 0 0 1 2 2 2
  spline S163 degree 2 poles (10.0218, -21.94) (9.9489, -21.94) (9.787, -22.0319) (9.7111, -22.1034) knots 0 0 0 1 2 2 2
  line L150 (9.7111, -22.1034) -> (9.7111, -23.1128)
  line L151 (9.7111, -23.1128) -> (9.4836, -23.1128)
  line L152 (9.4836, -23.1128) -> (9.4836, -21.762)
  line L153 (9.4836, -21.762) -> (9.7111, -21.762)
  line L154 (9.7111, -21.762) -> (9.7111, -21.9108)
  spline S164 degree 2 poles (9.7111, -21.9108) (9.8001, -21.8218) (9.9751, -21.7241) (10.0801, -21.7241) knots 0 0 0 1 2 2 2
  spline S165 degree 2 poles (10.0801, -21.7241) (10.1998, -21.7241) (10.385, -21.8335) (10.4331, -21.9575) knots 0 0 0 1 2 2 2
  spline S166 degree 2 poles (10.4331, -21.9575) (10.5367, -21.8423) (10.7322, -21.7241) (10.8459, -21.7241) knots 0 0 0 1 2 2 2
  spline S167 degree 2 poles (10.8459, -21.7241) (10.9335, -21.7241) (11.0764, -21.7781) (11.1289, -21.8393) knots 0 0 0 1 2 2 2
  spline S168 degree 2 poles (11.1289, -21.8393) (11.1829, -21.9006) (11.2427, -22.0844) (11.2427, -22.223) knots 0 0 0 1 2 2 2
  line L155 (11.2427, -22.223) -> (11.2427, -23.1128)
  line L156 (11.2427, -23.1128) -> (11.0152, -23.1128)
  line L157 (12.767, -23.4745) -> (11.3784, -23.4745)
  line L158 (11.3784, -23.4745) -> (11.3784, -23.3184)
  line L159 (11.3784, -23.3184) -> (12.767, -23.3184)
  line L160 (12.767, -23.3184) -> (12.767, -23.4745)
  line L161 (13.9733, -21.762) -> (13.4643, -23.1128)
  line L162 (13.4643, -23.1128) -> (13.26, -23.1128)
  line L163 (13.26, -23.1128) -> (12.7553, -21.762)
  line L164 (12.7553, -21.762) -> (13.0019, -21.762)
  line L165 (13.0019, -21.762) -> (13.3709, -22.8021)
  line L166 (13.3709, -22.8021) -> (13.737, -21.762)
  line L167 (13.737, -21.762) -> (13.9733, -21.762)
  line L168 (15.1315, -23.1128) -> (14.2534, -23.1128)
  line L169 (14.2534, -23.1128) -> (14.2534, -22.929)
  line L170 (14.2534, -22.929) -> (14.5801, -22.929)
  line L171 (14.5801, -22.929) -> (14.5801, -21.7227)
  line L172 (14.5801, -21.7227) -> (14.2534, -21.7227)
  line L173 (14.2534, -21.7227) -> (14.2534, -21.5578)
  spline S169 degree 2 poles (14.2534, -21.5578) (14.4387, -21.5578) (14.6137, -21.4528) (14.6254, -21.3069) knots 0 0 0 1 2 2 2
  line L174 (14.6254, -21.3069) -> (14.8121, -21.3069)
  line L175 (14.8121, -21.3069) -> (14.8121, -22.929)
  line L176 (14.8121, -22.929) -> (15.1315, -22.929)
  line L177 (15.1315, -22.929) -> (15.1315, -23.1128)
  dimension "d46" = 35
  constraints: 4 end point, 2 midpoint, 1 coincident, 1 collinear, 1 vertical, 1 vertical alignment, 4 other
extrude "Extrusion7" cut sketch "Sketch8" against normal blind 0.35 contours L6 L7 S0 S1 S2 S3 S4 S5 S6 L8 L9 L10 | L12 L13 L14 L15 | L16 L17 L18 L19 | S11 L20 L21 S12 S13 S14 S15 S16 S17 S18 S19 S20 L22 L23 S21 S22 S23 S24 S25 S26 S27 | S28 L24 L25 S29 S30 S31 S32 S33 S34 S35 S36 S37 L26 L27 S38 S39 S40 S41 S42 S43 S44 | S45 S46 S47 S48 L28 L29 S49 S50 S51 L30 L31 S52 S53 | S58 S59 S60 S61 S62 L33 L34 S63 S64 S65 S66 S67 L35 L36 S68 S69 | S70 L37 L38 L39 L40 L41 L42 L43 L44 L45 L46 L47 S71 S72 S73 L48 L49 S74 | L50 L51 L52 L53 | L54 L55 L56 L57 | S75 S76 S77 S78 | L58 L59 S83 S84 S85 L60 L61 L62 L63 L64 S86 S87 L65 | L66 L67 L68 L69 | S88 S89 L70 L71 L72 L73 L74 S90 S91 | L76 L77 L78 L79 | S96 S97 S98 S99 S100 S101 L80 S102 S103 S104 L81 L82 S105 S106 S107 L83 L84 L85 | S112 L87 L88 L89 L90 L91 L92 L93 L94 L95 L96 L97 S113 S114 S115 L98 L99 S116 | L100 S117 S118 L101 L102 L103 L104 L105 L106 L107 L108 L109 L110 L111 S119 S120 L112 | S121 S122 S123 S124 | L113 S129 S130 L114 L115 L116 L117 L118 S131 S132 L119 | L120 S133 S134 S135 S136 L121 L122 L123 S137 S138 S139 L124 L125 L126 L127 L128 S140 S141 S142 S143 S144 L129 L130 | L131 L132 L133 L134 | L135 S145 S146 S147 S148 L136 L137 L138 S149 S150 S151 L139 L140 L141 L142 L143 S152 S153 S154 S155 S156 L144 L145 | L146 S157 S158 S159 S160 L147 L148 L149 S161 S162 S163 L150 L151 L152 L153 L154 S164 S165 S166 S167 S168 L155 L156 | L157 L158 L159 L160 | L161 L162 L163 L164 L165 L166 L167 | L168 L169 L170 L171 L172 L173 S169 L174 L175 L176 L177
body "Solid1"
